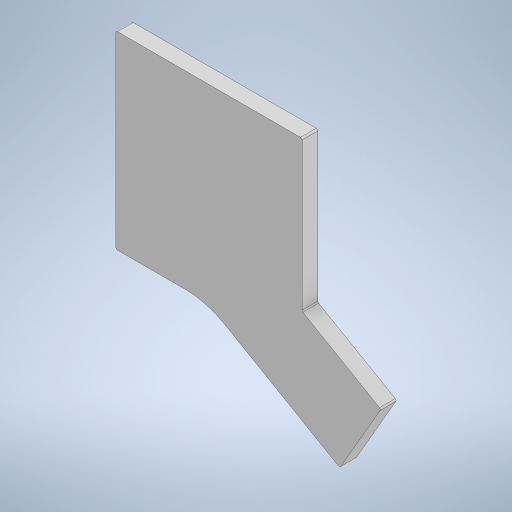
# Autodesk Inventor part: board-profile
Saved by Autodesk Inventor 2024.1 (Build 281209000, 209)
## iProperties
Created: 2023-11-01
Part Number: board-profile
Material: Générique
Document SubType Name: Modeling
Designer: Thibault
Density: 1 g/cm^3
Appearance: Par défaut
Author: Thibault
Autodesk Inventor part; units mm, degrees
ref_plane "YZ Plane" through (0, 0, 0) normal (1, 0, 0) x (0, 1, 0)
ref_plane "XZ Plane" through (0, 0, 0) normal (0, 1, 0) x (-1, 0, 0)
ref_plane "XY Plane" through (0, 0, 0) normal (0, 0, 1) x (1, 0, 0)
sketch "Esquisse1" plane through (0, 0, 0) normal (0, 0, 1) x (1, 0, 0)
  line L0 (-416.7812, 308.0239) -> (-298.7812, 308.0239)
  line L1 (-298.7812, 308.0239) -> (-298.7812, 188.0239)
  line L2 (-298.7812, 188.0239) -> (-416.7812, 188.0239)
  line L3 (-416.7812, 188.0239) -> (-416.7812, 308.0239)
  line L4 (-359.48, 188.0239) -> (-274.7812, 139.1231)
  line L5 (-359.48, 188.0239) -> (-261.6783, 188.0239) construction
  line L6 (-274.7812, 139.1231) -> (-248.7812, 184.1564)
  line L7 (-248.7812, 184.1564) -> (-318.2303, 224.2528)
  point P0 (-298.7812, 213.0239)
  point P1 (-298.7812, 213.0239)
  dimension "d4" = 120
  dimension "d5" = 118
  dimension "d10" = 30
  dimension "d11" = 52
  dimension "d21" = 95
  dimension "d22" = 50
  constraints: 16 end point, 5 point on line, 3 perpendicular, 2 horizontal, 2 parallel, 1 equal length
  measures "d4" distance of L0.end L1.end
  measures "d5" distance of L0.start L0.end
  measures "d10" angle of L4 L5
  measures "d11" distance of L4.end L6.end
  measures "d21" distance from line of point (-298.781, 213.024) L0
  measures "d22" horizontal distance of L6.end point (-298.781, 213.024)
extrude "Extrusion2" add sketch "Esquisse1" along normal blind 10
fillet "Congé1" radius 50 1 edges at (-359.48, 188.0239, 5)
fillet "Congé2" radius 1 1 edges at (-298.7812, 308.0239, 5)
fillet "Congé3" radius 1 1 edges at (-416.7812, 308.0239, 5)
fillet "Congé4" radius 1 1 edges at (-416.7812, 188.0239, 5)
fillet "Congé5" radius 1 1 edges at (-274.7812, 139.1231, 5)
fillet "Congé6" radius 1 2 edges at (-248.7812, 184.1564, 5) (-298.7812, 213.0239, 5)
